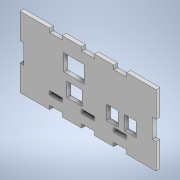
# Autodesk Inventor part: Стенка t3
Saved by Autodesk Inventor 2021 (Build 250183000, 183)
## iProperties
Created: 2021-04-11
Part Number: Стенка t3
Material: Типовые
Document SubType Name: Modeling
Designer: user
Density: 1 g/cm^3
Appearance: По умолчанию
Author: user
Autodesk Inventor part; units mm, degrees
ref_plane "YZ Plane" through (0, 0, 0) normal (1, 0, 0) x (0, 1, 0)
ref_plane "XZ Plane" through (0, 0, 0) normal (0, 1, 0) x (-1, 0, 0)
ref_plane "XY Plane" through (0, 0, 0) normal (0, 0, 1) x (1, 0, 0)
sketch "Эскиз1" plane through (0, 0, 0) normal (0, 0, 1) x (1, 0, 0)
  line L0 (-20, -22.5) -> (-20, -19.5)
  line L1 (-20, -19.5) -> (-30, -19.5)
  line L2 (-30, -19.5) -> (-30, -22.5)
  line L3 (0, -19.5) -> (-5, -19.5)
  line L4 (-5, -19.5) -> (-5, -22.5)
  line L5 (20, -22.5) -> (20, -19.5)
  line L6 (20, -19.5) -> (30, -19.5)
  line L7 (30, -19.5) -> (30, -22.5)
  line L8 (0, -19.5) -> (5, -19.5)
  line L9 (5, -19.5) -> (5, -22.5)
  line L10 (-53, 22.5) -> (-30, 22.5)
  line L11 (0, 19.5) -> (-5, 19.5)
  line L12 (-5, 19.5) -> (-5, 22.5)
  line L13 (-20, 22.5) -> (-5, 22.5)
  line L14 (-5, 22.5) -> (-20, 22.5)
  line L15 (-20, 22.5) -> (-20, 19.5)
  line L16 (-20, 19.5) -> (-30, 19.5)
  line L17 (-30, 19.5) -> (-30, 22.5)
  line L18 (-30, 22.5) -> (-53, 22.5)
  line L19 (0, 19.5) -> (5, 19.5)
  line L20 (5, 19.5) -> (5, 22.5)
  line L21 (20, 22.5) -> (20, 19.5)
  line L22 (20, 22.5) -> (5, 22.5)
  line L23 (5, 22.5) -> (20, 22.5)
  line L24 (20, 19.5) -> (30, 19.5)
  line L25 (30, 19.5) -> (30, 22.5)
  line L26 (53, 22.5) -> (30, 22.5)
  line L27 (30, 22.5) -> (53, 22.5)
  line L28 (-20, -32.5) -> (-20, -29.5)
  line L29 (-20, -29.5) -> (-30, -29.5)
  line L30 (-30, -29.5) -> (-30, -32.5)
  line L31 (5, -32.5) -> (5, -29.5)
  line L32 (5, -29.5) -> (-5, -29.5)
  line L33 (-5, -29.5) -> (-5, -32.5)
  line L34 (30, -32.5) -> (30, -29.5)
  line L35 (30, -29.5) -> (20, -29.5)
  line L36 (20, -29.5) -> (20, -32.5)
  line L37 (-30, -22.5) -> (-20, -22.5)
  line L38 (-5, -22.5) -> (5, -22.5)
  line L39 (20, -22.5) -> (30, -22.5)
  line L40 (-30, -32.5) -> (-53, -32.5)
  line L41 (-5, -32.5) -> (-20, -32.5)
  line L42 (53, -32.5) -> (30, -32.5)
  line L43 (20, -32.5) -> (5, -32.5)
  line L44 (-53, 2.5) -> (-50, 2.5)
  line L45 (-50, 2.5) -> (-50, -12.5)
  line L46 (-50, -12.5) -> (-53, -12.5)
  line L47 (53, 2.5) -> (50, 2.5)
  line L48 (50, 2.5) -> (50, -12.5)
  line L49 (50, -12.5) -> (53, -12.5)
  line L50 (-53, 22.5) -> (-53, 2.5)
  line L51 (-53, -12.5) -> (-53, -32.5)
  line L52 (53, -32.5) -> (53, -12.5)
  line L53 (53, 2.5) -> (53, 22.5)
  line L54 (-4.5, -17.529) -> (-4.5, -6.529)
  line L55 (-4.5, -6.529) -> (-16.5, -6.529)
  line L56 (-16.5, -6.529) -> (-16.5, -17.529)
  line L57 (26.5, -19.5) -> (23.5, -19.5)
  line L58 (14.5, -17.529) -> (14.5, -6.529)
  line L59 (14.5, -6.529) -> (23.5, -6.529)
  line L60 (23.5, -6.529) -> (23.5, -17.529)
  line L61 (-19, -1.5301) -> (-3, -1.5301)
  line L62 (-3, -1.5301) -> (-3, 11.4699)
  line L63 (-3, 11.4699) -> (-19, 11.4699)
  line L64 (-19, 11.4699) -> (-19, -1.5301)
  line L65 (-16.5, -6.529) -> (-16.5, -17.529)
  line L66 (-16.5, -17.529) -> (-4.5, -17.529)
  line L67 (14.5, -17.529) -> (23.5, -17.529)
  line L68 (28.5, -17.529) -> (37.5, -17.529)
  line L69 (37.5, -17.529) -> (37.5, -6.529)
  line L70 (37.5, -6.529) -> (28.5, -6.529)
  line L71 (28.5, -6.529) -> (28.5, -17.529)
  constraints: 144 end point, 18 equal length, 8 perpendicular, 5 horizontal
extrude "Выдавливание1" add sketch "Эскиз1" along normal blind 3
